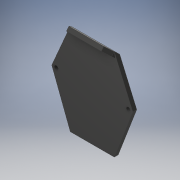
# Autodesk Inventor part: TARM08
Saved by Autodesk Inventor 2017 (Build 210142000, 142)
## iProperties
Created: 2018-10-22
Part Number: TARM08
Material: ABS Plastic
Document SubType Name: Modeling
Designer: Dell
Density: 1.06 g/cm^3
Appearance: Smooth - Black
Author: Dell
Autodesk Inventor part; units mm, degrees
ref_plane "YZ Plane" through (0, 0, 0) normal (1, 0, 0) x (0, 1, 0)
ref_plane "XZ Plane" through (0, 0, 0) normal (0, 1, 0) x (-1, 0, 0)
ref_plane "XY Plane" through (0, 0, 0) normal (0, 0, 1) x (1, 0, 0)
sketch "Sketch1" plane through (0, 0, 0) normal (0, 0, 1) x (1, 0, 0)
  line L0 (0, 0) -> (23.5818, 54.5446)
  line L1 (0, 0) -> (23.5818, -61.6289)
  line L2 (23.5818, -61.6289) -> (79.5818, -61.6289)
  line L3 (23.5818, 54.5446) -> (79.5818, 54.5446)
  line L4 (79.5818, 54.5446) -> (103.1637, 0)
  line L5 (103.1637, 0) -> (79.5818, -61.6289)
  circle A0 centre (5.7735, 0) radius 2.5
  circle A1 centre (97.3901, 0) radius 2.5
  dimension "d0" = 135.68
  dimension "d1" = 65.9865
  dimension "d2" = 59.424
  dimension "d3" = 56
  dimension "d4" = 65.9865
  dimension "d5" = 59.424
  dimension "d6" = 5
  dimension "d7" = 5
  dimension "d8" = 5.7735
  dimension "d9" = 5.7735
  constraints: 12 end point, 2 centre point, 2 horizontal, 2 horizontal alignment, 2 vertical alignment
  measures "d0" angle of L0 L1
  measures "d1" distance of L0.start L1.end
  measures "d2" distance of L0.start L0.end
  measures "d3" distance of L1.end L2.end
  measures "d4" distance of L4.end L2.end
  measures "d5" distance of L3.end L4.end
  measures "d6" diameter of A0
  measures "d7" diameter of A1
  measures "d8" distance of L4.end A1.centre
  measures "d9" distance of L0.start A0.centre
extrude "Extrusion1" add sketch "Sketch1" along normal blind 5
ref_plane "Work Plane2" through (23.5818, 54.5446, 5) normal (0, 0.7488345, -0.662757) x (-1, 0, 0)
sketch "Sketch3" plane through (23.5818, 54.5446, 5) normal (0, 0.7488345, -0.662757) x (-1, 0, 0)
  ellipse E0 centre (-73.8083, -39.894) end of major axis (-71.3083, -39.894) minor radius 1.6569 projected
  ellipse E1 centre (17.8083, -39.894) end of major axis (20.3083, -39.894) minor radius 1.6569 projected
  line L0 (23.5818, -39.894) -> (0, -3.7442) projected
  line L1 (0, -3.7442) -> (-56, -3.7442) projected
  line L2 (-56, -3.7442) -> (-79.5818, -39.894) projected
  line L3 (-79.5818, -39.894) -> (-56, -80.7389) projected
  line L4 (-56, -80.7389) -> (0, -80.7389) projected
  line L5 (0, -80.7389) -> (23.5818, -39.894) projected
  line L6 (-56, -3.7442) -> (-79.5818, -39.894) projected
  line L7 (-56, -3.7442) -> (-56, 0) projected
  line L8 (-79.5818, -36.1498) -> (-56, 0) projected
  line L9 (-79.5818, -39.894) -> (-79.5818, -36.1498) projected
  line L10 (0, -3.7442) -> (-56, -3.7442) projected
  line L11 (0, -3.7442) -> (0, 0) projected
  line L12 (-56, 0) -> (0, 0) projected
  line L13 (-56, -3.7442) -> (-56, 0) projected
  line L14 (0, 0) -> (23.5818, -36.1498) projected
  line L15 (23.5818, -39.894) -> (0, -3.7442) projected
  line L16 (23.5818, -39.894) -> (23.5818, -36.1498) projected
  line L17 (0, 0) -> (23.5818, -36.1498) projected
  line L18 (0, -3.7442) -> (0, 0) projected
  constraints: 2 other
extrude "Extrusion2" cut sketch "Sketch3" along normal through all contours E0 | E1 | L5 L4 L3 L2 L1 L0 | L0 L11 L14 L16 | L1 L7 L12 L11 | L2 L9 L8 L7
sketch "Sketch4" plane through (23.5818, 54.5446, 5) normal (0, 0.7488345, -0.662757) x (1, 0, 0)
  line L0 (56, 0) -> (0, 0) projected
  line L1 (56, 0) -> (50.2265, -10)
  line L2 (50.2265, -10) -> (5.7735, -10)
  line L3 (5.7735, -10) -> (0, 0)
  line L4 (57.9132, 6.677) -> (56, 0) projected
  line L5 (79.5818, 36.1498) -> (56, 0) projected
  line L6 (79.5818, 39.894) -> (79.5818, 36.1498) projected
  line L7 (57.9132, 6.677) -> (79.5818, 39.894) projected
  line L8 (0, 0) -> (-1.9132, 6.677) projected
  line L9 (56, 0) -> (0, 0) projected
  line L10 (57.9132, 6.677) -> (56, 0) projected
  line L11 (-1.9132, 6.677) -> (57.9132, 6.677) projected
  line L12 (0, 0) -> (-1.9132, 6.677) projected
  line L13 (-23.5818, 39.894) -> (-1.9132, 6.677) projected
  line L14 (-23.5818, 39.894) -> (-23.5818, 36.1498) projected
  line L15 (0, 0) -> (-23.5818, 36.1498) projected
  dimension "d16" = 60
  dimension "d17" = 60
  dimension "d18" = 10
  constraints: 6 end point, 1 parallel
  measures "d16" angle of L1 L0
  measures "d17" angle of L0 L3
  measures "d18" distance between parallel lines of L0 L2
extrude "Extrusion3" add sketch "Sketch4" against normal blind 5 contours L1 L2 L3 L0 | L0 L8 L11 L4
equation "\"d4\" = d1"
equation "\"d5\" = d2"
body "Solid1"
